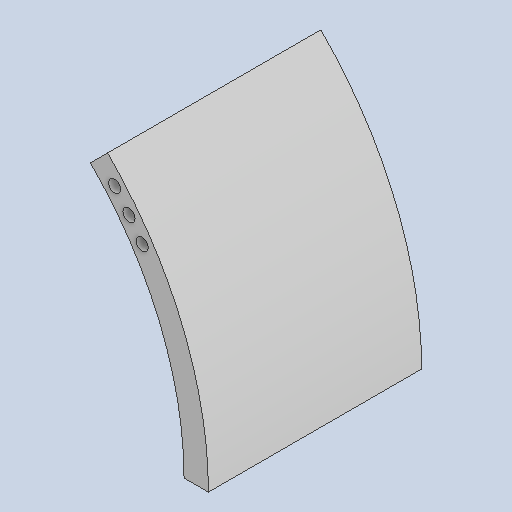
# Autodesk Inventor part: HoodGearSmooth
Saved by Autodesk Inventor 2023 (Build 270158000, 158)
## iProperties
Created: 2023-11-15
Part Number: HoodGearSmooth
Material: Generic
Document SubType Name: Modeling
Designer: jackc
Density: 1 g/cm^3
Appearance: Default
Author: jackc
Autodesk Inventor part; units mm, degrees
ref_plane "YZ Plane" through (0, 0, 0) normal (1, 0, 0) x (0, 1, 0)
ref_plane "XZ Plane" through (0, 0, 0) normal (0, 1, 0) x (-1, 0, 0)
ref_plane "XY Plane" through (0, 0, 0) normal (0, 0, 1) x (1, 0, 0)
sketch "Sketch1" plane through (0, 0, 0) normal (0, 0, 1) x (1, 0, 0)
  arc A0 (287.02, 0) -> (202.9538, 202.9538) centre (0, 0) ccw
  arc A1 (266.7, 0) -> (188.5854, 188.5854) centre (0, 0) ccw
  line L0 (202.9538, 202.9538) -> (188.5854, 188.5854)
  line L1 (266.7, 0) -> (287.02, 0)
  line L2 (188.5854, 188.5854) -> (0, 0) construction
  dimension "d1" = 266.7
  dimension "d5" = 287.02
  dimension "d6" = 45
  constraints: 6 end point, 4 point on circle, 2 centre point, 1 coincident, 1 collinear, 1 concentric, 1 horizontal, 1 horizontal alignment
  measures "d1" radius of A1
  measures "d5" radius of A0
  measures "d6" angle of L1 L2
extrude "Extrusion1" add sketch "Sketch1" along normal blind 177.8
sketch "Sketch2" plane through (0, 0, 177.8) normal (0, 0, 1) x (1, 0, 0)
  line L0 (287.02, 0) -> (266.7, 0) projected
  line L1 (188.5854, 188.5854) -> (202.9538, 202.9538) projected
  arc A0 (276.86, 0) -> (195.7696, 195.7696) centre (0, 0) ccw construction
  arc A1 (188.5854, 188.5854) -> (266.7, 0) centre (0, 0) ccw projected
  circle A2 centre (208.776, 181.8352) radius 5.0625
  circle A3 centre (220.786, 167.048) radius 5.0625
  circle A4 centre (231.7506, 151.4698) radius 5.0625
  dimension "d7" = 10.125
  dimension "d8" = 19.05
  dimension "d9" = 19.05
  dimension "d10" = 19.05
  constraints: 5 point on circle, 4 centre point, 2 equal radius, 2 midpoint, 1 concentric
  measures "d7" diameter of A2
  measures "d8" distance from line of L1 A2.centre
  measures "d9" distance of A3.centre A2.centre
  measures "d10" distance of A3.centre A4.centre
extrude "Extrusion2" cut sketch "Sketch2" against normal blind 177.8
equation "\"d1\" = BallSize + 0.5 * WheelSize - Compression"
equation "\"WheelSize1\" = 101.6"
equation "\"BallSize1\" = 304.8"
equation "\"Compression1\" = 12.7"
equation "\"BallSize\" = 228.6"
equation "\"WheelSize\" = 101.6"
equation "\"Compression\" = 12.7"
body "Solid1"
